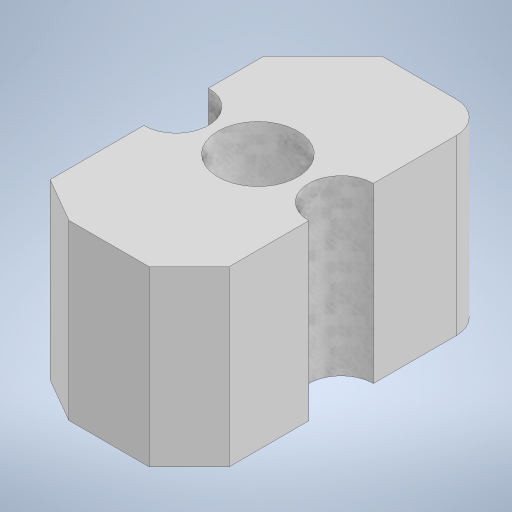
# Autodesk Inventor part: Part2
Saved by Autodesk Inventor 2023 (Build 270158000, 158)
## iProperties
Created: 2022-07-14
Part Number: Part2
Material: Generic
Document SubType Name: Modeling
Designer: earls
Density: 1 g/cm^3
Appearance: Default
Author: earls
Autodesk Inventor part; units mm, degrees
ref_plane "YZ Plane" through (0, 0, 0) normal (1, 0, 0) x (0, 1, 0)
ref_plane "XZ Plane" through (0, 0, 0) normal (0, 1, 0) x (-1, 0, 0)
ref_plane "XY Plane" through (0, 0, 0) normal (0, 0, 1) x (1, 0, 0)
sketch "Sketch1" plane through (0, 0, 0) normal (0, 0, 1) x (1, 0, 0)
  point P0 (0, 0)
sketch "Sketch2" plane through (0, 0, 0) normal (0, 1, 0) x (-1, 0, 0)
  line L0 (18.3793, 32.1145) -> (-18.6207, 32.1145)
  line L1 (-18.6207, 32.1145) -> (-18.6207, -28.8855)
  line L2 (-18.6207, -28.8855) -> (18.3793, -28.8855)
  line L3 (18.3793, -28.8855) -> (18.3793, 32.1145)
  line L4 (-18.6207, 32.1145) -> (-18.6207, 28.0145)
  line L5 (-18.6207, 28.0145) -> (-14.5207, 28.0145)
  line L6 (-14.5207, 28.0145) -> (-7.6207, 28.0145)
  line L7 (-7.6207, 28.0145) -> (6.2793, 28.0145)
  line L8 (6.2793, 28.0145) -> (14.2793, 28.0145) construction
  line L9 (14.0338, 32.3374) -> (14.0338, 23.5374)
  line L10 (6.2793, 28.0145) -> (14.0338, 23.5374)
  line L11 (14.0338, 23.5374) -> (14.0338, 7.3145)
  arc A0 (14.0338, 7.3145) -> (14.0338, -3.8855) centre (14.0338, 1.7145) ccw
  line L12 (14.0338, -3.8855) -> (14.0338, -13.4855)
  arc A1 (-14.5207, -3.8855) -> (-14.5207, 7.3145) centre (-14.5207, 1.7145) ccw
  line L13 (-14.5207, -3.8855) -> (-14.5207, -18.1855)
  line L14 (-7.6207, 28.0145) -> (-14.5207, 21.1145)
  line L15 (-14.5207, 32.1145) -> (-14.5207, 28.0145)
  line L16 (-14.5207, 21.1145) -> (-14.5207, 7.3145)
  line L17 (-14.5207, -18.1855) -> (-14.5207, -23.6855) construction
  line L18 (-14.5207, -23.6855) -> (3.8338, -23.6855)
  line L19 (14.0338, -13.4855) -> (3.8338, -23.6855)
  line L20 (-1.3662, -28.8855) -> (-1.8697, -29.389)
  arc A2 (-14.5207, -18.1855) -> (-9.0207, -23.6855) centre (-9.0207, -18.1855) ccw
  line L21 (14.0338, 1.7145) -> (-14.5207, 1.7145)
  circle A3 centre (-0.1207, 1.7145) radius 6.9
  point P0 (0, 0)
  dimension "d2" = 37
  dimension "d3" = 61
  dimension "d4" = 4.1
  dimension "d5" = 4.1
  dimension "d6" = 6.9
  dimension "d7" = 13.9
  dimension "d9" = 8.8
  dimension "d10" = 30
  dimension "d12" = 30.4
  dimension "d13" = 24.8
  dimension "d14" = 45.6
  dimension "d16" = 24.8
  dimension "d17" = 30.4
  dimension "d20" = 50.3
  dimension "d21" = 45
  dimension "d22" = 5.5
  dimension "d24" = 5.5
  dimension "d25" = 5.5
  dimension "d26" = 18.5
  dimension "d27" = 13.8
  constraints: 44 end point, 7 point on line, 7 vertical, 6 point on circle, 5 coincident, 4 centre point, 4 horizontal, 3 perpendicular, 2 parallel
  measures "d2" distance of L2.end L1.end
  measures "d3" distance of L1.end L0.end
  measures "d4" distance of L0.end L4.end
  measures "d5" distance of L4.end L5.end
  measures "d6" distance of L5.end L6.end
  measures "d7" distance of L7.start L7.end
  measures "d9" distance of L9.start L9.end
  measures "d10" angle of L10 L8
  measures "d12" distance from line of point (14.034, 1.715) L0
  measures "d13" distance from line of L11.end L0
  measures "d14" distance from line of L12.end L0
  measures "d16" distance of L15.start L16.end
  measures "d17" distance of point (-14.521, 1.715) L15.start
  measures "d20" distance of L13.end L15.start
  measures "d21" angle of L14 L6
  measures "d22" distance of L13.end L17.end
  measures "d24" distance from line of A2.end L17
  measures "d25" radius of A2
  measures "d26" distance from line of point (-0.121, 1.715) L3
  measures "d27" diameter of A3
extrude "Extrusion1" add sketch "Sketch2" along normal blind 30 contours L11 A0 L21 A3 A1 L16 L14 L7 L10 | A0 L12 L19 L18 A2 L13 A1 L21 A3
body "Solid1"
